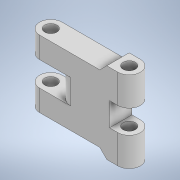
# Autodesk Inventor part: short_link_v2
Saved by Autodesk Inventor 2022 (Build 260153000, 153)
## iProperties
Created: 2022-05-21
Part Number: short_link_v2
Material: Generic
Document SubType Name: Modeling
Designer: kylem
Density: 1 g/cm^3
Appearance: Default
Author: kylem
Autodesk Inventor part; units mm, degrees
sketch "Sketch1" plane through (0, 0, 0) normal (0, 1, 0) x (-1, 0, 0)
  line L0 (0, 0) -> (18, 0)
  line L1 (18, 0) -> (18, -4)
  line L2 (18, -4) -> (0, -4)
  line L3 (0, -4) -> (0, 0)
  line L4 (18, -2) -> (16, -2)
  line L5 (9, -4) -> (9, -3)
  circle A0 centre (16, -2) radius 1.1
  circle A1 centre (2, -2) radius 1.1
  dimension "d0" = 18
  dimension "d1" = 4
  dimension "d2" = 2
  dimension "d3" = 2.2
  constraints: 12 end point, 2 centre point, 2 horizontal, 2 midpoint, 2 parallel, 1 coincident, 1 perpendicular, 1 symmetric about line, 1 vertical, 1 other
  measures "d0" distance of L1.end L2.end
  measures "d1" distance of L0.end L1.end
  measures "d2" distance of L4.start L4.end
  measures "d3" diameter of A0
sketch "Sketch1 outline for Extrusion1" plane through (0, 0, 0) normal (0, 1, 0) x (-1, 0, 0)
  line L0 (18, -4) -> (18, 0)
  line L1 (0, -4) -> (18, -4)
  line L2 (0, 0) -> (0, -4)
  line L3 (18, 0) -> (0, 0)
extrude "Extrusion1" add sketch "Sketch1 outline for Extrusion1" along normal blind 8
sketch "Sketch2" plane through (0, 0, -4) normal (0, 0, -1) x (-1, 0, 0)
  line L0 (18, 0) -> (18, 8) projected
  line L1 (18, 8) -> (18, 6.1)
  line L2 (18, 0) -> (0, 0) projected
  line L3 (18, 0) -> (18, 1.9)
  line L4 (18, 6.1) -> (14.5, 6.1)
  line L5 (14.5, 6.1) -> (14.5, 1.9)
  line L6 (14.5, 1.9) -> (18, 1.9)
  line L7 (18, 1.9) -> (18, 6.1)
  dimension "d6" = 1.9
  dimension "d7" = 1.9
  dimension "d8" = 3.5
  constraints: 12 end point, 2 parallel, 2 point on line, 1 horizontal, 1 perpendicular
  measures "d6" distance of L0.end L1.end
  measures "d7" distance of L0.start L3.end
  measures "d8" distance of L6.end L5.end
sketch "Sketch2 outline for Extrusion2" plane through (0, 0, -4) normal (0, 0, -1) x (-1, 0, 0)
  line L0 (14.5, 6.1) -> (14.5, 1.9)
  line L1 (18, 6.1) -> (14.5, 6.1)
  line L2 (18, 1.9) -> (18, 6.1)
  line L3 (14.5, 1.9) -> (18, 1.9)
extrude "Extrusion2" cut sketch "Sketch2 outline for Extrusion2" against normal blind 8
ref_plane "Work Plane1" through (-9, 0, 0) normal (1, 0, 0) x (0, 0, -1)
mirror "Mirror1" about plane through (-9, 0, 0) normal (1, 0, 0) of "Extrusion2"
sketch "Sketch1 outline for Extrusion3" plane through (0, 0, 0) normal (0, 1, 0) x (-1, 0, 0)
  circle A0 centre (2, -2) radius 1.1
  circle A1 centre (16, -2) radius 1.1
extrude "Extrusion3" cut sketch "Sketch1 outline for Extrusion3" along normal blind 8
sketch "Sketch4" plane through (0, 8, 0) normal (0, 1, 0) x (1, 0, 0)
  line L0 (-18, 0) -> (0, 0) projected
  line L1 (0, 0) -> (-4, 0)
  line L2 (-4, 0) -> (-4, 4)
  line L3 (-4, 4) -> (0, 4)
  line L4 (0, 4) -> (0, 0)
  circle A0 centre (-2, 2) radius 1.1 projected
  circle A1 centre (-2, 2) radius 1.1
  dimension "d14" = 4
  dimension "d15" = 4
  dimension "d16" = 2.2
  constraints: 8 end point, 2 parallel, 1 centre point, 1 coincident, 1 horizontal, 1 perpendicular
  measures "d14" distance of L2.end L3.end
  measures "d15" distance of L1.end L2.end
  measures "d16" diameter of A1
sketch "Sketch4 outline for Extrusion4" plane through (0, 8, 0) normal (0, 1, 0) x (1, 0, 0)
  line L0 (0, 0) -> (0, 4)
  line L1 (-4, 0) -> (0, 0)
  line L2 (0, 4) -> (-4, 4)
  line L3 (-4, 4) -> (-4, 0)
  circle A0 centre (-2, 2) radius 1.1
extrude "Extrusion4" add sketch "Sketch4 outline for Extrusion4" along normal blind 3.25
ref_plane "Work Plane2" through (-3.5, 4, 0) normal (0, 1, 0) x (1, 0, 0)
mirror "Mirror2" about plane through (-3.5, 4, 0) normal (0, 1, 0) of "Extrusion4"
fillet "Fillet2" radius 2 8 edges at (0, 8.675, -4) (0, -0.675, -4) (0, -0.675, 0) (0, 8.675, 0) (-18, 7.05, -4) (-18, 0.95, -4) (-18, 7.05, 0) (-18, 0.95, 0)
chamfer "Chamfer1" distance 3.25 angle 45 2 edges at (-4, 8, -2) (-4, 0, -2)
sketch "Sketch5" plane through (-14.5, 1.9, 0) normal (0, 0, 1) x (1, 0, 0)
  line L0 (0, 4.2) -> (0, 0) projected
  line L1 (0, 4.2) -> (2, 4.2)
  line L2 (2, 4.2) -> (2, 0)
  line L3 (2, 0) -> (0, 0)
  line L4 (0, 0) -> (0, 4.2)
  point P0 (14.5, -1.9)
  point P1 (0, 0)
  dimension "d23" = 2
  constraints: 8 end point, 2 parallel, 1 horizontal, 1 perpendicular
  measures "d23" distance of L2.end L3.end
sketch "Sketch5 outline for Extrusion5" plane through (-14.5, 1.9, 0) normal (0, 0, 1) x (1, 0, 0)
  line L0 (0, 0) -> (2, 0)
  line L1 (0, 4.2) -> (0, 0)
  line L2 (2, 4.2) -> (0, 4.2)
  line L3 (2, 0) -> (2, 4.2)
extrude "Extrusion5" cut sketch "Sketch5 outline for Extrusion5" against normal blind 20
sketch "Sketch6" plane through (0, 8, 0) normal (0, 1, 0) x (1, 0, 0)
  line L0 (-7.25, 4) -> (-4, 4) projected
  line L1 (-16, 0) -> (-12.5, 0) projected
  line L2 (-7.25, 4) -> (-16, 4)
  line L3 (-16, 4) -> (-16, 0)
  line L4 (-16, 0) -> (-7.25, 0)
  line L5 (-7.25, 0) -> (-7.25, 4)
  circle A0 centre (-16, 2) radius 2
  circle A1 centre (-16, 2) radius 1.1
  point P0 (0, 0)
  constraints: 8 end point, 2 parallel, 1 centre point, 1 coincident, 1 horizontal, 1 midpoint, 1 perpendicular, 3 other
sketch "Sketch6 outline for Extrusion6" plane through (0, 8, 0) normal (0, 1, 0) x (1, 0, 0)
  arc A0 (-16, 4) -> (-16, 0) centre (-16, 2) ccw
  line L0 (-7.25, 4) -> (-16, 4)
  line L1 (-16, 0) -> (-12.5, 0)
  line L2 (-7.25, 0) -> (-7.25, 4)
  line L3 (-12.5, 0) -> (-7.25, 0)
  circle A1 centre (-16, 2) radius 1.1
extrude "Extrusion6" add sketch "Sketch6 outline for Extrusion6" along normal blind 2
sketch "Sketch7" plane through (-3.5, 1.9, -4) normal (0, 0, -1) x (-1, 0, 0)
  line L0 (3.75, 6.1) -> (3.75, 8.1)
  line L1 (3.75, 8.1) -> (1.311143, 8.1)
  line L2 (1.311143, 8.1) -> (1.311143, 4.926567)
  line L3 (1.311143, 4.926567) -> (3.75, 4.926567)
  line L4 (3.75, 4.926567) -> (3.75, 8.1)
  point P0 (-3.5, -1.9)
  constraints: 8 end point, 2 parallel, 1 horizontal, 1 perpendicular
sketch "Sketch7 outline for Extrusion7" plane through (-3.5, 1.9, -4) normal (0, 0, -1) x (-1, 0, 0)
  line L0 (1.311143, 4.926567) -> (3.75, 4.926567)
  line L1 (1.311143, 8.1) -> (1.311143, 4.926567)
  line L2 (3.75, 8.1) -> (1.311143, 8.1)
  line L3 (3.75, 6.1) -> (3.75, 8.1)
  line L4 (3.75, 4.926567) -> (3.75, 6.1)
extrude "Extrusion7" add sketch "Sketch7 outline for Extrusion7" against normal blind 4
ref_plane "Work Plane3" through (0, 4, 0) normal (0, 1, 0) x (1, 0, 0)
mirror "Mirror3" about plane through (0, 4, 0) normal (0, 1, 0) of "Extrusion6", "Extrusion7"
sketch "Sketch8" plane through (-3.5, 1.9, -4) normal (0, 0, -1) x (-1, 0, 0)
  line L0 (12.5, 0) -> (14.5, 0)
  line L1 (14.5, 0) -> (14.5, -0.1)
  line L2 (14.5, -3.9) -> (14.5, 0)
  line L3 (14.5, -0.1) -> (8.337258, -0.1)
  line L4 (14.5, 4.2) -> (12.5, 4.2)
  line L5 (14.5, 4.2) -> (14.5, 4.3)
  line L6 (14.5, 4.2) -> (14.5, 8.1)
  line L7 (14.5, 4.3) -> (6.488775, 4.3)
  line L8 (14.5, -0.1) -> (9.5, -0.1)
  line L9 (9.5, -0.1) -> (9.5, 4.3)
  line L10 (9.5, 4.3) -> (14.5, 4.3)
  line L11 (14.5, 4.3) -> (14.5, -0.1)
  point P0 (-3.5, -1.9)
  point P1 (9.5, -0.1)
  dimension "d30" = 0.1
  dimension "d31" = 0.1
  constraints: 16 end point, 3 perpendicular, 3 point on line, 2 parallel, 1 horizontal
  measures "d30" distance of L0.end L1.end
  measures "d31" distance of L4.start L5.end
sketch "Sketch8 outline for Extrusion8" plane through (-3.5, 1.9, -4) normal (0, 0, -1) x (-1, 0, 0)
  line L0 (14.5, 0) -> (14.5, 4.2)
  line L1 (14.5, -0.1) -> (14.5, 0)
  line L2 (9.5, -0.1) -> (14.5, -0.1)
  line L3 (9.5, 4.3) -> (9.5, -0.1)
  line L4 (14.5, 4.3) -> (9.5, 4.3)
  line L5 (14.5, 4.2) -> (14.5, 4.3)
extrude "Extrusion8" cut sketch "Sketch8 outline for Extrusion8" against normal blind 4
sketch "Sketch9" plane through (-3.5, 1.9, -4) normal (0, 0, -1) x (-1, 0, 0)
  line L0 (12.5, -0.1) -> (9.5, -0.1) projected
  line L1 (9, 0) -> (9, 4.2) projected
  line L2 (9.5, -0.1) -> (9, -0.1)
  line L3 (9, -0.1) -> (9, 0)
  line L4 (9, 0) -> (9.5, 0)
  line L5 (9.5, 0) -> (9.5, -0.1)
  line L6 (9, 4.2) -> (9.5, 4.2) projected
  line L7 (9.5, 4.2) -> (9.5, 4.3) projected
  line L8 (9, 4.2) -> (9.5, 4.2)
  line L9 (9.5, 4.2) -> (9.5, 4.3)
  line L10 (9.5, 4.3) -> (9, 4.3)
  line L11 (9, 4.3) -> (9, 4.2)
  point P0 (-3.5, -1.9)
  constraints: 16 end point, 4 parallel, 2 horizontal, 2 perpendicular
sketch "Sketch9 outline for Extrusion9" plane through (-3.5, 1.9, -4) normal (0, 0, -1) x (-1, 0, 0)
  line L0 (9, 4.3) -> (9, 4.2)
  line L1 (9.5, 4.3) -> (9, 4.3)
  line L2 (9.5, 4.2) -> (9.5, 4.3)
  line L3 (9, 4.2) -> (9.5, 4.2)
  line L4 (9, 0) -> (9, -0.1)
  line L5 (9.5, 0) -> (9, 0)
  line L6 (9.5, -0.1) -> (9.5, 0)
  line L7 (9, -0.1) -> (9.5, -0.1)
extrude "Extrusion9" cut sketch "Sketch9 outline for Extrusion9" against normal blind 20
fillet "Fillet3" radius 2 2 edges at (-12.5, 4, -4) (-12.5, 4, 0)
body "Solid1"
